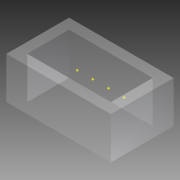
# Autodesk Inventor part: CrimpSocket
Saved by Autodesk Inventor 2012 (Build 160160000, 160)
## iProperties
Created: 2014-07-20
Part Number: CrimpSocket
Material: Default
Document SubType Name: Modeling
Designer: Anon
Density: 1 g/cm^3
Categories: <MemberInstance><Categories><Category DisplayName="" Mnemonic="CABLEANDHARNESS" InternalName="e4a7e005-5e42-4d16-b293-125e7f0d0512"><Category DisplayName="" Mnemonic="CONNECTORS" InternalName="6f634eba-a678-4820-a31d-2c2d5ee6728e"><CategoryParameter DisplayName="" Mnemonic="REFDES" InternalName="c3740e8c-60ab-4d5d-8584-52b73222f2f0"/><Category DisplayName="" Mnemonic="RIBBONCABLE" InternalName="27621a3d-53ec-49ed-8225-e2ac65e8eb52"/></Category></Category></Categories><FamilyTemplate><FamilyTemplateParameters></FamilyTemplateParameters></FamilyTemplate><CategoryParameterMap><ParamToTemplateMap><ParamToTemplate CategoryParameter="//CategoryParameter[@InternalName='c3740e8c-60ab-4d5d-8584-52b73222f2f0']" ConstantValue=""/></ParamToTemplateMap></CategoryParameterMap></MemberInstance>
Author: Anon
Autodesk Inventor part; units mm, degrees
ref_plane "YZ Plane" through (0, 0, 0) normal (1, 0, 0) x (0, 1, 0)
ref_plane "XZ Plane" through (0, 0, 0) normal (0, 1, 0) x (-1, 0, 0)
sketch "Sketch1" plane through (0, 0, 0) normal (0, 0, 1) x (1, 0, 0)
  line L0 (-4, 2) -> (4, 2)
  line L1 (4, 2) -> (4, -2)
  line L2 (4, -2) -> (-4, -2)
  line L3 (-4, -2) -> (-4, 2)
  line L4 (5, 3) -> (-5, 3)
  line L5 (-5, 3) -> (-5, -3)
  line L6 (-5, -3) -> (5, -3)
  line L7 (5, -3) -> (5, 3)
  point P0 (0, 0)
  dimension "d0" = 8
  dimension "d1" = 4
  dimension "d2" = 2
  dimension "d3" = 4
  dimension "d5" = 1
  constraints: 16 end point, 4 parallel, 2 perpendicular, 1 horizontal, 3 other
  measures "d0" distance between parallel lines of L1 L3
  measures "d1" distance from line of point (0, 0) L3
  measures "d2" distance from line of point (0, 0) L0
  measures "d3" distance between parallel lines of L0 L2
  measures "d5" distance between parallel lines of L4 L0
extrude "Extrusion1" add sketch "Sketch1" along normal blind 4
ref_plane "Work Plane1" through (0, 0, 2) normal (0, 0, 1) x (1, 0, 0)
sketch "Sketch2" plane through (0, 0, 2) normal (0, 0, 1) x (1, 0, 0)
  line L0 (0, 0) -> (5.4411, 0) construction
  point P0 (2.25, 1)
  point P1 (0.75, 1)
  point P2 (-0.75, 1)
  point P3 (-2.25, 1)
  dimension "d11" = 1.5
  dimension "d16" = 2.25
  dimension "d17" = 1
  constraints: 2 end point, 2 horizontal, 3 other
  measures "d11" distance of point (2.25, 1) point (0.75, 1)
  measures "d16" horizontal distance of L0.start point (2.25, 1)
  measures "d17" vertical distance of point (-0.75, 1) L0.start
body "Solid1"
